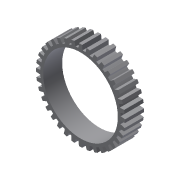
# Autodesk Inventor part: 200_Holder_Lambdaplate_1
Saved by Autodesk Inventor 2019 (Build 230136000, 136)
## iProperties
Created: 2019-07-08
Part Number: 200_Holder_Lambdaplate_1
Material: Generic
Document SubType Name: Modeling
Designer: diederichbenedict
Density: 1 g/cm^3
Appearance: Default
Author: diederichbenedict
Autodesk Inventor part; units mm, degrees
ref_plane "YZ Plane" through (0, 0, 0) normal (1, 0, 0) x (0, 1, 0)
ref_plane "XZ Plane" through (0, 0, 0) normal (0, 1, 0) x (-1, 0, 0)
sketch "Sketch6" plane through (0, 0, 0) normal (0, 0, 1) x (1, 0, 0)
  circle A0 centre (0, 0) radius 12.5 projected
  circle A1 centre (0, 0) radius 12.8
  circle A2 centre (0, 0) radius 13.8
  dimension "d32" = 0.3
  dimension "d33" = 1
  constraints: 2 centre point
  measures "d32" radial gap between concentric circles of A0 A1
  measures "d33" radial gap between concentric circles of A1 A2
ref_plane "Work Plane1" through (-12.5, -12.5, 6.5) normal (0, 0, 1) x (1, 0, 0)
extrude "Extrusion4" add sketch "Sketch6" along normal up to surface (6.5 mm away) contours A2
sketch "Sketch7" plane through (0, 0, 0) normal (0, 0, -1) x (-1, 0, 0)
  line L0 (13.8, 0) -> (0, 0)
  line L1 (0, 0) -> (0, 0)
  line L2 (0, 0) -> (13.7811, -0.7222)
  line L3 (0, 0) -> (0, 0) construction
  line L4 (0, 0) -> (0, 0) construction
  line L5 (0, 0) -> (0, 0) construction
  line L6 (13.7811, -0.7222) -> (15.279, -0.8007) construction
  line L7 (15.2834, -0.7222) -> (15.2834, 0)
  line L8 (15.2834, 0) -> (13.8, 0)
  line L9 (13.7811, -0.7222) -> (15.2834, -0.7222)
  circle A0 centre (0, 0) radius 13.8 construction
  line L10 (13.7811, 0.7222) -> (15.279, 0.8007) construction
  line L11 (15.2834, 0.7222) -> (15.2834, 0)
  line L12 (13.7811, 0.7222) -> (15.2834, 0.7222)
  line L13 (13.7811, -0.7222) -> (15.2834, -0.5378)
  line L14 (13.7811, -0.7222) -> (15.2947, -0.7222) construction
  line L15 (13.7811, 0.7222) -> (15.2834, 0.5378)
  line L16 (13.7811, 0.7222) -> (15.2947, 0.7222) construction
  line L17 (15.2834, 0.5378) -> (15.2834, -0.5378)
  line L18 (13.7811, -0.7222) -> (13.7811, 0.7222)
  dimension "d37" = 0
  dimension "d38" = 1.5
  dimension "d44" = 3
  dimension "d45" = 7
  dimension "d46" = 7
  constraints: 38 end point, 4 horizontal, 3 collinear, 3 equal length, 3 perpendicular, 3 symmetric about line, 2 point on circle, 2 point on line, 2 vertical, 1 midpoint
  measures "d37" distance between parallel lines of L4 L2
  measures "d38" distance of L2.end L6.end
  measures "d44" angle of L0 L2
  measures "d45" angle of L14 L13
  measures "d46" angle of L15 L16
extrude "Extrusion5" add sketch "Sketch7" against normal up to surface (6.5 mm away) contours L8 L7 L13 L18 L0 | L0 L18 L15 L11 L8
pattern_circular "Circular Pattern2" count 36 over 360 about axis through (0, 0, 0) along (0, 0, 1) of "Extrusion5"
body "Solid2"
